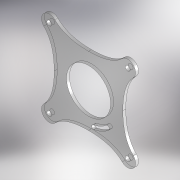
# Autodesk Inventor part: YawBottomPlate
Saved by Autodesk Inventor 2018.2 (Build 222227000, 227)
## iProperties
Created: 2018-03-25
Part Number: YawBottomPlate
Material: Generic
Document SubType Name: Modeling
Designer: mansu
Density: 1 g/cm^3
Appearance: Clear Clear
Mass: 12.9156 g
Surface Area: 104.57 cm^2
Volume: 12.9156 cm^3
Author: mansu
Autodesk Inventor part; units mm, degrees
ref_plane "YZ Plane" through (0, 0, 0) normal (1, 0, 0) x (0, 1, 0)
ref_plane "XZ Plane" through (0, 0, 0) normal (0, 1, 0) x (-1, 0, 0)
ref_plane "XY Plane" through (0, 0, 0) normal (0, 0, 1) x (1, 0, 0)
sketch "Sketch1" plane through (0, 0, 0) normal (0, 1, 0) x (-1, 0, 0)
  line L0 (40, -40) -> (-40, -40) construction
  line L1 (-40, -40) -> (-40, 40) construction
  line L2 (-40, 40) -> (40, 40) construction
  line L3 (40, 40) -> (40, -40) construction
  line L4 (40, -40) -> (-40, 40) construction
  line L5 (-40, -40) -> (40, 40) construction
  circle A0 centre (-40, -40) radius 2.5
  arc A1 (-45.6569, -34.3431) -> (-34.3431, -45.6569) centre (-40, -40) ccw
  line L6 (-45.6569, -34.3431) -> (-35, -23.6863) construction
  line L7 (-35, -23.6863) -> (-35, 0) construction
  spline S0 degree 2 poles (-45.6569, -34.3431) (-35, -23.6863) (-35, 0) knots 1 1 1 2 2 2
  line L8 (-34.3431, -45.6569) -> (-45.6569, -34.3431) construction
  circle A2 centre (0, 0) radius 22.5
  line L9 (-34.3431, -45.6569) -> (-23.6863, -35) construction
  line L10 (-23.6863, -35) -> (0, -35) construction
  spline S1 degree 2 poles (-34.3431, -45.6569) (-23.6863, -35) (0, -35) knots 1 1 1 2 2 2
  line L11 (0, 0) -> (0, -47.3827) construction
  line L12 (0, 0) -> (-76.4691, 0) construction
  circle A3 centre (-40, 40) radius 2.5
  arc A4 (-34.3431, 45.6569) -> (-45.6569, 34.3431) centre (-40, 40) ccw
  line L13 (-45.6569, 34.3431) -> (-35, 23.6863) construction
  line L14 (-35, 23.6863) -> (-35, 0) construction
  spline S2 degree 2 poles (-45.6569, 34.3431) (-35, 23.6863) (-35, 0) knots 1 1 1 2 2 2
  spline S3 degree 2 poles (-34.3431, 45.6569) (-23.6863, 35) (0, 35) knots 1 1 1 2 2 2
  line L15 (-34.3431, 45.6569) -> (-23.6863, 35) construction
  line L16 (-23.6863, 35) -> (0, 35) construction
  circle A5 centre (40, -40) radius 2.5
  arc A6 (34.3431, -45.6569) -> (45.6569, -34.3431) centre (40, -40) ccw
  line L17 (45.6569, -34.3431) -> (35, -23.6863) construction
  line L18 (35, -23.6863) -> (35, 0) construction
  spline S4 degree 2 poles (45.6569, -34.3431) (35, -23.6863) (35, 0) knots 1 1 1 2 2 2
  spline S5 degree 2 poles (34.3431, -45.6569) (23.6863, -35) (0, -35) knots 1 1 1 2 2 2
  line L19 (34.3431, -45.6569) -> (23.6863, -35) construction
  line L20 (23.6863, -35) -> (0, -35) construction
  spline S6 degree 2 poles (45.6569, 34.3431) (35, 23.6863) (35, 0) knots 1 1 1 2 2 2
  arc A7 (45.6569, 34.3431) -> (34.3431, 45.6569) centre (40, 40) ccw
  circle A8 centre (40, 40) radius 2.5
  spline S7 degree 2 poles (34.3431, 45.6569) (23.6863, 35) (0, 35) knots 1 1 1 2 2 2
  line L21 (45.6569, 34.3431) -> (35, 23.6863) construction
  line L22 (35, 23.6863) -> (35, 0) construction
  line L23 (34.3431, 45.6569) -> (23.6863, 35) construction
  line L24 (23.6863, 35) -> (0, 35) construction
  dimension "d0" = 80
  dimension "d1" = 80
  dimension "d2" = 5
  dimension "d4" = 45
  dimension "d5" = 5
  dimension "d6" = 45
  dimension "d7" = 8
  constraints: 22 symmetric about line, 18 end point, 9 centre point, 8 point on circle, 4 midpoint, 2 coincident, 2 horizontal, 2 parallel, 2 vertical, 1 concentric, 1 horizontal alignment, 1 perpendicular, 1 tangent, 30 other
  measures "d0" distance of L1.end L2.end
  measures "d1" distance of L0.end L1.end
  measures "d2" diameter of A0
  measures "d4" angle of L0 L6
  measures "d5" distance between parallel lines of L1 L7
  measures "d6" diameter of A2
  measures "d7" radius of A1
extrude "Extrusion1" add sketch "Sketch1" along normal blind 3
sketch "Sketch2" plane through (0, 3, 0) normal (0, 1, 0) x (1, 0, 0)
  arc A0 (21.2132, 21.2132) -> (7.7646, 28.9778) centre (0, 0) ccw construction
  arc A1 (22.6274, 22.6274) -> (8.2822, 30.9096) centre (0, 0) ccw
  arc A2 (19.799, 19.799) -> (7.2469, 27.0459) centre (0, 0) ccw
  arc A3 (19.799, 19.799) -> (22.6274, 22.6274) centre (21.2132, 21.2132) ccw
  arc A4 (8.2822, 30.9096) -> (7.2469, 27.0459) centre (7.7646, 28.9778) ccw
  line L0 (0, 0) -> (21.2132, 21.2132) construction
  line L1 (0, 0) -> (7.7646, 28.9778) construction
  line L2 (0, 0) -> (0, 28.9934) construction
  dimension "d10" = 30
  dimension "d11" = 4
  dimension "d12" = 30
  dimension "d15" = 15
  constraints: 10 point on circle, 6 end point, 5 centre point, 4 tangent, 1 coincident, 1 vertical
  measures "d10" angle of L0 L1
  measures "d11" diameter of A3
  measures "d12" radius of A0
  measures "d15" angle of L2 L1
extrude "Extrusion2" cut sketch "Sketch2" against normal up to next
body "Solid1"
